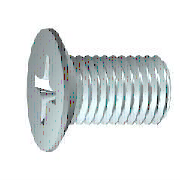
# Autodesk Inventor part: ANSI B18.6.3 - 1/4-20 x 3/4
Saved by Autodesk Inventor 2022 Beta2 (Build 260130000, 130) ContinuousBuild 0
## iProperties
Created: 2006-01-18
Part Number: ANSI B18.6.3 - 1/4-20 x 3/4
Material: Steel, Mild
Description: Countersunk Flat Head Screw
Vendor: Autodesk Inc.
Document SubType Name: Modeling
Standard: ANSI B18.6.3
Designer: PMiller
Standards Organization: ANSI
Language: en-US
Size Designation: 1/4-20 x 3/4
Categories: <MemberInstance Version="R10.0.0"><Categories><Category DisplayName="Fasteners" InternalName="e4da775c-781d-43d5-af7c-5136215cf5a6" Mnemonic="FSTN"><Category DisplayName="Bolts" InternalName="536e6df0-f778-49ac-b2f2-25c71d2aa0b2" Mnemonic="SCRW"><CategoryParameter DisplayName="Nominal Diameter" InternalName="8bbe3f8e-44cf-40a9-a251-3a6edc8168d6" Mnemonic="nomdia" /><CategoryParameter DisplayName="Nominal Length" InternalName="238ecbaf-3e6c-45dd-aa95-4068c8e0fd02" Mnemonic="nomlen" /><CategoryParameter DisplayName="Thread Series Designation" InternalName="87c5849c-b3a5-4c3e-9c9b-2feecef9be86" Mnemonic="thrserdsgn" /><CategoryParameter DisplayName="Thread Class" InternalName="ebc0d23b-2cc6-4d2a-b376-d52aae53bab6" Mnemonic="thrclss" /><CategoryParameter DisplayName="Thread Designation" InternalName="586d5e89-370a-4089-914f-0110033585c7" Mnemonic="thrdesign" /><CategoryParameter DisplayName="Threads per Unit" InternalName="bdc6e7d2-ffd0-4d9c-a173-16b95ebb912d" Mnemonic="thrperunit1" /><CategoryParameter DisplayName="Thread Pitch" InternalName="bb82302e-82d8-4176-8fc1-c5d7bb17d5ad" Mnemonic="pitch1" /><CategoryParameter DisplayName="Nominal Diameter Designation" InternalName="03caf894-eafd-4c09-a035-916ac084b87b" Mnemonic="nomdiadesig" /><Category DisplayName="Countersunk" InternalName="49656530-5684-4604-a233-68d537625f23" Mnemonic="CSSCRW"><CategoryParameter DisplayName="Shank Diameter" InternalName="7ece923f-d8ee-40d5-83f8-980cad520964" Mnemonic="grpdia" /><CategoryParameter DisplayName="Grip Length" InternalName="2fff3de5-ce2a-45fd-9425-99ddc9dff352" Mnemonic="grplen" /><CategoryParameter DisplayName="Thread Length" InternalName="207f0278-6dec-43ab-bffc-1c6d03e64de4" Mnemonic="thrlen" /><CategoryParameter DisplayName="Head Diameter" InternalName="a509cd31-06d1-44c5-b54e-d7a695352906" Mnemonic="headdia" /><CategoryParameter DisplayName="Head Height" InternalName="57526df9-da71-45fb-acb4-1d0529a34778" Mnemonic="headh" /><CategoryParameter DisplayName="Head Angle" InternalName="dbcfc1e0-7990-403e-bc2e-90d1c639222a" Mnemonic="headang" /><CategoryParameter DisplayName="Property Class" InternalName="5249b721-5ecc-4781-a2e8-d7e3bda3ecca" Mnemonic="propclss" /></Category></Category></Category></Categories><FamilyTemplate Id="sc0002.ipt"><FamilyTemplateParameters><FamilyTemplateParameter ValueType="xs:double" Id="1" ObjectReferenceKey="NND" ObjectType="kUserParameterObject" /><FamilyTemplateParameter ValueType="xs:double" Id="2" ObjectReferenceKey="NLG" ObjectType="kUserParameterObject" /><FamilyTemplateParameter ValueType="xs:double" Id="3" ObjectReferenceKey="GEL" ObjectType="kUserParameterObject" /><FamilyTemplateParameter ValueType="xs:double" Id="4" ObjectReferenceKey="KOH" ObjectType="kUserParameterObject" /><FamilyTemplateParameter ValueType="xs:double" Id="5" ObjectReferenceKey="KOD" ObjectType="kUserParameterObject" /><FamilyTemplateParameter ValueType="xs:double" Id="6" ObjectReferenceKey="SBR" ObjectType="kUserParameterObject" /><FamilyTemplateParameter ValueType="xs:double" Id="7" ObjectReferenceKey="INTI" ObjectType="kUserParameterObject" /><FamilyTemplateParameter ValueType="xs:double" Id="8" ObjectReferenceKey="SDM" ObjectType="kUserParameterObject" /><FamilyTemplateParameter ValueType="xs:double" Id="9" ObjectReferenceKey="GAL" ObjectType="kUserParameterObject" /><FamilyTemplateParameter ValueType="xs:double" Id="10" ObjectReferenceKey="SPD" ObjectType="kUserParameterObject" /><FamilyTemplateParameter ValueType="xs:double" Id="11" ObjectReferenceKey="GD" ObjectType="kUserParameterObject" /><FamilyTemplateParameter ValueType="xs:double" Id="12" ObjectReferenceKey="GD1" ObjectType="kUserParameterObject" /><FamilyTemplateParameter ValueType="xs:double" Id="13" ObjectReferenceKey="EPV" ObjectType="kUserParameterObject" /><FamilyTemplateParameter ValueType="xs:double" Id="14" ObjectReferenceKey="GUL" ObjectType="kUserParameterObject" /><FamilyTemplateParameter ValueType="xs:double" Id="15" ObjectReferenceKey="BDM" ObjectType="kUserParameterObject" /><FamilyTemplateParameter ValueType="xs:double" Id="16" ObjectReferenceKey="SEWI" ObjectType="kUserParameterObject" /><FamilyTemplateParameter ValueType="xs:double" Id="17" ObjectReferenceKey="THREADDIA" ObjectType="kUserParameterObject" /><FamilyTemplateParameter ValueType="xs:string" Id="18" ObjectReferenceKey="TPU" ObjectType="kUserParameterObject" /><FamilyTemplateParameter ValueType="xs:double" Id="19" ObjectReferenceKey="PTC" ObjectType="kUserParameterObject" /><FamilyTemplateParameter ValueType="xs:double" Id="20" ObjectReferenceKey="TOA" ObjectType="kUserParameterObject" /></FamilyTemplateParameters></FamilyTemplate><CategoryParameterMap><ParamToTemplateMap><ParamToTemplate CategoryParameter="//CategoryParameter[@InternalName='bb82302e-82d8-4176-8fc1-c5d7bb17d5ad']" TemplateParameter="19" /><ParamToTemplate CategoryParameter="//CategoryParameter[@InternalName='207f0278-6dec-43ab-bffc-1c6d03e64de4']" TemplateParameter="3" /><ParamToTemplate CategoryParameter="//CategoryParameter[@InternalName='87c5849c-b3a5-4c3e-9c9b-2feecef9be86']" ConstantValue="UNC" /><ParamToTemplate CategoryParameter="//CategoryParameter[@InternalName='03caf894-eafd-4c09-a035-916ac084b87b']" ConstantValue="1/4" /><ParamToTemplate CategoryParameter="//CategoryParameter[@InternalName='ebc0d23b-2cc6-4d2a-b376-d52aae53bab6']" ConstantValue="2A" /><ParamToTemplate CategoryParameter="//CategoryParameter[@InternalName='57526df9-da71-45fb-acb4-1d0529a34778']" TemplateParameter="4" /><ParamToTemplate CategoryParameter="//CategoryParameter[@InternalName='8bbe3f8e-44cf-40a9-a251-3a6edc8168d6']" TemplateParameter="1" /><ParamToTemplate CategoryParameter="//CategoryParameter[@InternalName='bdc6e7d2-ffd0-4d9c-a173-16b95ebb912d']" TemplateParameter="18" /><ParamToTemplate CategoryParameter="//CategoryParameter[@InternalName='dbcfc1e0-7990-403e-bc2e-90d1c639222a']" TemplateParameter="16" /><ParamToTemplate CategoryParameter="//CategoryParameter[@InternalName='a509cd31-06d1-44c5-b54e-d7a695352906']" TemplateParameter="5" /><ParamToTemplate CategoryParameter="//CategoryParameter[@InternalName='586d5e89-370a-4089-914f-0110033585c7']" ConstantValue="1/4-20 UNC" /><ParamToTemplate CategoryParameter="//CategoryParameter[@InternalName='238ecbaf-3e6c-45dd-aa95-4068c8e0fd02']" TemplateParameter="2" /><ParamToTemplate CategoryParameter="//CategoryParameter[@InternalName='2fff3de5-ce2a-45fd-9425-99ddc9dff352']" ConstantValue="0.75-0.472" /><ParamToTemplate CategoryParameter="//CategoryParameter[@InternalName='7ece923f-d8ee-40d5-83f8-980cad520964']" TemplateParameter="11" /></ParamToTemplateMap></CategoryParameterMap></MemberInstance>
Density: 1 g/cm^3
Appearance: Steel
Author: PMiller
Autodesk Inventor part; units mm, degrees
ref_plane "YZ Plane" through (0, 0, 0) normal (1, 0, 0) x (0, 1, 0)
ref_plane "XZ Plane" through (0, 0, 0) normal (0, 1, 0) x (-1, 0, 0)
ref_plane "XY Plane" through (0, 0, 0) normal (0, 0, 1) x (1, 0, 0)
sketch "Sketch1" plane through (0, 0, 0) normal (0, 0, 1) x (1, 0, 0)
  line L0 (4.3434, 0) -> (19.05, 0)
  line L1 (19.05, 0) -> (19.05, 3.175)
  line L2 (19.05, 3.175) -> (3.8862, 3.175)
  line L3 (0.8289, 5.7404) -> (0, 5.7404)
  line L4 (-1.905, 0) -> (24.765, 0) projected
  line L5 (0, -0.574) -> (0, 7.4625) projected
  line L6 (0, 3.5941) -> (3.3098, 1.9439)
  line L7 (3.3098, 1.9439) -> (4.3434, 0)
  line L8 (3.8862, 3.175) -> (0.8289, 5.7404)
  line L9 (0, 5.7404) -> (0, 3.5941)
  dimension "d2" = 6.35
  dimension "d3" = 11.4808
  dimension "d4" = 4.3434
  dimension "d5" = 7.1882
  dimension "d6" = 26.5
  dimension "d7" = 62
  dimension "d13" = 40
  dimension "d14" = 3.8862
  dimension "d15" = 19.05
  constraints: 16 end point, 3 parallel, 2 point on line, 1 collinear, 1 horizontal, 1 perpendicular
  measures "d2" diameter of L2 L0
  measures "d3" diameter of L3 L0
  measures "d4" distance from line of L0.start L5
  measures "d5" diameter of L6.start L0
  measures "d6" angle of L6 L0
  measures "d7" angle of L7 L0
  measures "d13" angle of L8 L0
  measures "d14" distance from line of L2.end L5
  measures "d15" distance between parallel lines of L1 L5
revolve "Body" add sketch "Sketch1" angle 360 about axis through (4.3434, 0, 0) along (1, 0, 0) contours L7 L6 L5 L3 L8 L2 L1 L0
sketch "Sketch2" plane through (0, 0, 0) normal (-1, 0, 0) x (0, 0, 1)
  line L0 (0, -6.8885) -> (0, 9.1846) projected
  line L1 (-6.8885, 0) -> (9.1846, 0) projected
  line L2 (0, 3.5941) -> (0, 0) construction
  line L3 (0, 0) -> (3.5941, 0) construction
  arc A0 (1.198, 0) -> (0, 1.198) centre (0, 0) ccw
  line L4 (0, 0) -> (0.7947, 0.7947) construction
  arc A1 (1.797, 0) -> (0, 1.7971) centre (0, 0) ccw construction
  line L5 (0.4572, 3.5649) -> (0.4751, 1.7331)
  line L6 (3.5649, 0.4572) -> (1.7331, 0.4751)
  arc A2 (0.4751, 1.7331) -> (1.7331, 0.4751) centre (1.7455, 1.7455) ccw
  arc A3 (3.5941, 0) -> (3.5649, 0.4572) centre (0, 0) ccw
  arc A4 (0.4572, 3.5649) -> (0, 3.5941) centre (0, 0) ccw
  arc A5 (3.5649, 0.4572) -> (0.4572, 3.5649) centre (0, 0) ccw
  line L7 (0.4572, -3.5649) -> (0.4751, -1.7331)
  line L8 (3.5649, -0.4572) -> (1.7331, -0.4751)
  arc A6 (1.7331, -0.4751) -> (0.4751, -1.7331) centre (1.7455, -1.7455) ccw
  arc A7 (3.5649, -0.4572) -> (3.5941, 0) centre (0, 0) ccw
  arc A8 (0, -3.5941) -> (0.4572, -3.5649) centre (0, 0) ccw
  arc A9 (0.4572, -3.5649) -> (3.5649, -0.4572) centre (0, 0) ccw
  line L9 (-0.4572, 3.5649) -> (-0.4751, 1.7331)
  line L10 (-3.5649, 0.4572) -> (-1.7331, 0.4751)
  arc A10 (-1.7331, 0.4751) -> (-0.4751, 1.7331) centre (-1.7455, 1.7455) ccw
  arc A11 (-3.5649, 0.4572) -> (-3.5941, 0) centre (0, 0) ccw
  arc A12 (0, 3.5941) -> (-0.4572, 3.5649) centre (0, 0) ccw
  arc A13 (-0.4572, 3.5649) -> (-3.5649, 0.4572) centre (0, 0) ccw
  arc A14 (-3.5649, -0.4572) -> (-0.4572, -3.5649) centre (0, 0) ccw
  arc A15 (-0.4572, -3.5649) -> (0, -3.5941) centre (0, 0) ccw
  arc A16 (-3.5941, 0) -> (-3.5649, -0.4572) centre (0, 0) ccw
  line L11 (-3.5649, -0.4572) -> (-1.7331, -0.4751)
  arc A17 (-0.4751, -1.7331) -> (-1.7331, -0.4751) centre (-1.7455, -1.7455) ccw
  line L12 (-0.4572, -3.5649) -> (-0.4751, -1.7331)
  dimension "d18" = 45
  dimension "d19" = 2.3961
  dimension "d20" = 3.5941
  dimension "d21" = 7.1882
  dimension "d22" = 0.4572
  constraints: 37 point on circle, 22 end point, 19 symmetric about line, 18 centre point, 4 coincident, 3 tangent, 2 collinear, 2 midpoint, 2 perpendicular, 2 point on line, 19 other
  measures "d18" angle of L4 L3
  measures "d19" diameter of A0
  measures "d20" diameter of A1
  measures "d21" diameter of A5
  measures "d22" distance from line of L5.start L2
extrude "Slot" add sketch "Sketch2" against normal up to next draft 5 contours A2 L5 A5 L6 | L9 A10 L10 A13 | L7 A6 L8 A9 | A14 L11 A17 L12
fillet "Fillet1" radius 0.1829 4 edges at (0, 3.5941, 0) (0, 0, 3.5941) (0, -3.5941, 0) (0, 0, -3.5941)
thread "Thread" size "1/4-20 UNC" class "2A" standard "ANSI Unified Screw Threads" length 11.9888
chamfer "Chamfer1" distance 0.9525 distance2 0.9525 1 edges at (19.05, -3.175, 0) measured on face at (19.05, -0.3658, -0.0841)
equation "\"d2\" = GD"
equation "\"d3\" = KOD"
equation "\"d4\" = INTI"
equation "\"d5\" = SDM"
equation "\"d13\" = 0.5 * SEWI"
equation "\"d14\" = KOH"
equation "\"d15\" = NLG"
equation "\"d19\" = 0.333333 * SDM"
equation "\"d20\" = 0.5 * SDM"
equation "\"d21\" = SDM"
equation "\"d22\" = 0.5 * SBR"
equation "\"d45\" = INTI"
equation "\"d25\" = 0.2 * SBR"
equation "\"d9\" = GEL"
equation "\"d11\" = -0.5 * SPD + 0.5 * GD"
equation "\"d12\" = GUL"
equation "\"GD\" = NND"
equation "\"NLG\" = 19.05"
equation "\"GEL\" = 11.9888"
equation "\"KOD\" = 11.4808"
equation "\"KOH\" = 3.8862"
equation "\"SDM\" = 7.1882"
equation "\"INTI\" = 4.3434"
equation "\"SBR\" = 0.9144"
equation "\"GUL\" = 0.75 * GAL"
equation "\"SPD\" = 4.445"
equation "\"SEWI\" = 80deg"
equation "\"d0\" = NLG"
equation "\"d1\" = KOH"
equation "\"d17\" = SDM"
equation "\"NND\" = 6.35"
equation "\"GAL\" = 1.27"
equation "\"GD1\" = SPD"
equation "\"BDM\" = NND"
equation "\"THREADDIA\" = 6.35"
equation "\"TOA\" = 30deg"
body "Solid1"
